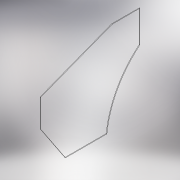
# Autodesk Inventor part: end_plate
Saved by Autodesk Inventor 2018.2 (Build 222227000, 227)
## iProperties
Created: 2017-10-22
Part Number: end_plate
Material: CFRP
Document SubType Name: Modeling
Designer: ku_sk
Density: 1.43 g/cm^3
Appearance: カーボンファイバー
Mass: 2260.49 g
Surface Area: 6541.63 cm^2
Volume: 1580.77 cm^3
Author: ku_sk
Autodesk Inventor part; units mm, degrees
ref_plane "YZ Plane" through (0, 0, 0) normal (1, 0, 0) x (0, 1, 0)
ref_plane "XZ Plane" through (0, 0, 0) normal (0, 1, 0) x (-1, 0, 0)
ref_plane "XY Plane" through (0, 0, 0) normal (0, 0, 1) x (1, 0, 0)
sketch "スケッチ1" plane through (0, 0, 0) normal (1, 0, 0) x (0, 1, 0)
  line L0 (-670, 240) -> (-670, 540)
  line L1 (-670, 540) -> (-400, 720)
  line L2 (-400, 720) -> (-200, 720)
  line L3 (-200, 720) -> (0, 200)
  line L4 (0, 200) -> (0, 0)
  line L5 (0, 0) -> (-230, 0)
  arc A0 (-230, 0) -> (-670, 240) centre (-746.431, -423.4569) ccw
  dimension "d0" = 720
  dimension "d1" = 300
  dimension "d2" = 180
  dimension "d3" = 270
  dimension "d4" = 200
  dimension "d5" = 670
  dimension "d6" = 230
  dimension "d7" = 200
  constraints: 12 end point, 2 perpendicular, 2 point on circle, 1 centre point, 1 coincident, 1 horizontal, 1 parallel
  measures "d0" distance between parallel lines of L5 L2
  measures "d1" distance of L0.start L0.end
  measures "d2" distance from line of L0.end L2
  measures "d3" distance from line of L1.end L0
  measures "d4" distance of L3.end L4.end
  measures "d5" distance between parallel lines of L0 L4
  measures "d6" distance of L4.end L5.end
  measures "d7" distance of L1.end L2.end
extrude "押し出し1" add sketch "スケッチ1" along normal blind 5
